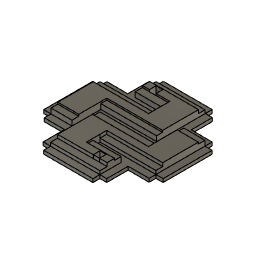
PythonKeyChain (Autodesk Fusion 360 design; units mm, degrees)
Autodesk Fusion 360 part; units mm, degrees
sketch "pythonSketch" plane through (0, 0, 0) normal (0, 0, 1) x (1, 0, 0)
  line L0 (12.2612, -2.5668) -> (26.7, -2.5668)
  line L1 (26.7, -2.5668) -> (26.7, -4.6)
  line L2 (26.7, -4.6) -> (28.8, -4.6)
  line L3 (28.8, -4.6) -> (28.8, -10.8729)
  line L4 (28.8, -10.8729) -> (35, -10.8729)
  line L5 (35, -10.8729) -> (35, -13)
  line L6 (35, -13) -> (37.1372, -13)
  line L7 (37.1372, -13) -> (37.1372, -27.5)
  line L8 (37.1372, -27.5) -> (35, -27.5)
  line L9 (35, -27.5) -> (35, -29.5)
  line L10 (35, -29.5) -> (28.7977, -29.5)
  line L11 (28.7977, -29.5) -> (28.7977, -35.8264)
  line L12 (28.7977, -35.8264) -> (26.777, -35.8264)
  line L13 (26.777, -35.8264) -> (26.777, -37.8923)
  line L14 (26.777, -37.8923) -> (12.2101, -37.8923)
  line L15 (12.2101, -37.8923) -> (12.2101, -35.8264)
  line L16 (12.2101, -35.8264) -> (10, -35.8264)
  line L17 (10, -35.8264) -> (10, -29.5)
  line L18 (10, -29.5) -> (4, -29.5)
  line L19 (4, -29.5) -> (4, -27.5)
  line L20 (4, -27.5) -> (1.8353, -27.5)
  line L21 (1.8353, -27.5) -> (1.8353, -13)
  line L22 (1.8353, -13) -> (4, -13)
  line L23 (4, -13) -> (4, -11)
  line L24 (4, -11) -> (10.1818, -11)
  line L25 (10.1818, -11) -> (10.1818, -4.699)
  line L26 (10.1818, -4.699) -> (12.2719, -4.699)
  line L27 (12.2719, -4.699) -> (12.2612, -2.5668)
  line L28 (20.3394, -10.8945) -> (20.3377, -12.9134)
  line L29 (20.3377, -12.9134) -> (4, -13)
  line L30 (4, -13) -> (4, -27.5)
  line L31 (12.2719, -4.699) -> (26.7, -4.699)
  line L32 (26.7, -4.699) -> (26.7, -19)
  line L33 (26.7, -19) -> (10.2082, -19)
  line L34 (10.2082, -19) -> (10.2082, -27.5)
  line L35 (10.2082, -27.5) -> (4, -27.5)
  line L36 (35, -13) -> (28.7314, -13)
  line L37 (28.7314, -13) -> (28.7314, -21.2454)
  line L38 (28.7314, -21.2454) -> (12.2026, -21.2454)
  line L39 (12.2101, -35.8264) -> (26.777, -35.8264)
  line L40 (26.777, -29.5705) -> (18.4403, -29.5705)
  line L41 (18.4403, -29.5705) -> (18.4403, -27.4588)
  line L42 (18.4403, -27.4588) -> (35, -27.5)
  line L43 (26.777, -29.5705) -> (26.777, -35.8264)
  line L44 (35, -13) -> (35, -27.5)
  line L45 (14.3261, -6.7876) -> (16.303, -6.7893)
  line L46 (16.303, -6.7893) -> (16.3013, -8.805)
  line L47 (16.3013, -8.805) -> (14.3448, -8.8033)
  line L48 (14.3448, -8.8033) -> (14.3261, -6.7876)
  line L49 (22.6655, -31.7169) -> (24.5, -31.7169)
  line L50 (24.5, -31.7169) -> (24.5, -33.682)
  line L51 (24.5, -33.682) -> (22.7033, -33.682)
  line L52 (22.7033, -33.682) -> (22.6655, -31.7169)
  line L53 (12.2703, -6.5992) -> (26.7, -6.5992)
  line L54 (26.7, -4.699) -> (12.2719, -4.699)
  line L55 (4, -15) -> (20.3439, -15)
  line L56 (20.3439, -15) -> (20.3377, -12.9134)
  line L57 (20.3377, -12.9134) -> (4, -13)
  line L58 (4, -13) -> (4, -15)
  line L59 (10.2082, -19) -> (10.2082, -17.2376)
  line L60 (10.2082, -17.2376) -> (26.7, -17.2376)
  line L61 (26.7, -19) -> (10.2082, -19)
  line L62 (26.7, -19) -> (26.7, -17.2376)
  line L63 (4, -25.5) -> (10.2082, -25.5)
  line L64 (10.2082, -25.5) -> (10.2082, -27.5)
  line L65 (10.2082, -27.5) -> (4, -27.5)
  line L66 (4, -27.5) -> (4, -25.5)
  line L67 (28.7314, -14.9455) -> (35, -14.9455)
  line L68 (35, -13) -> (28.7314, -13)
  line L69 (28.7314, -14.9455) -> (35, -14.9455)
  line L70 (12.2063, -23.4679) -> (28.77, -23.4594)
  line L71 (28.77, -23.4594) -> (28.7314, -21.2454)
  line L72 (28.7314, -21.2454) -> (12.2026, -21.2454)
  line L73 (12.2063, -23.4679) -> (12.2026, -21.2454)
  line L74 (18.4403, -27.4588) -> (18.4452, -25.4862)
  line L75 (18.4452, -25.4862) -> (35, -25.4862)
  line L76 (35, -25.4862) -> (35, -27.5)
  line L77 (35, -27.5) -> (18.4403, -27.4588)
  line L78 (18.4403, -29.5705) -> (18.4403, -31.5)
  line L79 (18.4403, -31.5) -> (26.777, -31.5)
  line L80 (26.777, -29.5705) -> (18.4403, -29.5705)
  line L81 (12.2101, -35.8264) -> (12.2101, -33.7534)
  line L82 (26.777, -33.682) -> (26.777, -35.8264)
  line L83 (12.2101, -35.8264) -> (12.2101, -33.7534)
  line L84 (12.2101, -35.8264) -> (12.2101, -33.7534)
  line L85 (12.2101, -33.7534) -> (26.777, -33.682)
  line L86 (26.777, -33.682) -> (26.777, -35.8264)
  line L87 (26.777, -35.8264) -> (12.2101, -35.8264)
  line L88 (12.2063, -23.4679) -> (12.2101, -33.7534)
  line L89 (12.2719, -4.699) -> (12.2703, -6.5992)
  line L90 (12.2666, -10.81) -> (12.2666, -10.8876)
  line L91 (12.2703, -6.5992) -> (12.2666, -10.8876)
  line L92 (20.3394, -10.8945) -> (12.2666, -10.8876)
  line L93 (20.3394, -10.8945) -> (20.3385, -11.904)
  line L94 (12.2684, -8.7434) -> (20.3394, -8.7503)
  line L95 (20.3394, -8.7503) -> (16.3039, -8.7468)
  line L96 (20.3394, -8.7503) -> (20.3394, -10.8945)
  constraint horizontal L0
  constraint perpendicular L0 L1
  constraint perpendicular L1 L2
  constraint perpendicular L2 L3
  constraint perpendicular L1 L4
  constraint perpendicular L4 L5
  constraint perpendicular L5 L6
  constraint perpendicular L6 L7
  constraint perpendicular L7 L8
  constraint perpendicular L8 L9
  constraint perpendicular L9 L10
  constraint perpendicular L10 L11
  constraint perpendicular L11 L12
  constraint perpendicular L12 L13
  constraint perpendicular L13 L14
  constraint perpendicular L12 L15
  constraint perpendicular L15 L16
  constraint perpendicular L16 L17
  constraint perpendicular L17 L18
  constraint perpendicular L16 L19
  constraint perpendicular L17 L20
  constraint perpendicular L20 L21
  constraint perpendicular L17 L22
  constraint perpendicular L22 L23
  constraint perpendicular L23 L24
  constraint perpendicular L22 L25
  constraint perpendicular L25 L26
  constraint perpendicular L20 L30
  constraint perpendicular L1 L31
  constraint perpendicular L31 L32
  constraint perpendicular L1 L33
  constraint perpendicular L33 L34
  constraint perpendicular L19 L35
  constraint perpendicular L5 L36
  constraint perpendicular L36 L37
  constraint perpendicular L5 L38
  constraint perpendicular L13 L39
  constraint perpendicular L13 L40
  constraint perpendicular L40 L41
  constraint perpendicular L12 L43
  constraint perpendicular L8 L44
  constraint perpendicular L45 L46
  constraint perpendicular L46 L47
  constraint horizontal L49
  constraint perpendicular L49 L50
  constraint perpendicular L50 L51
  constraint coincident L32 L53.end
  constraint perpendicular L32 L53
  constraint parallel L31 L54
  constraint coincident L90.start L89
  constraint coincident L30 L55.start
  constraint perpendicular L30 L55
  constraint parallel L29 L57
  constraint perpendicular L33 L59
  constraint coincident L32 L60.end
  constraint perpendicular L32 L60
  constraint coincident L30 L63.start
  constraint coincident L34 L63.end
  constraint perpendicular L34 L63
  constraint coincident L37 L67.start
  constraint coincident L44 L67.end
  constraint perpendicular L44 L67
  constraint parallel L38 L72
  constraint perpendicular L42 L74
  constraint coincident L44 L75.end
  constraint perpendicular L44 L75
  constraint parallel L42 L77
  constraint perpendicular L40 L78
  constraint coincident L43 L79.end
  constraint perpendicular L43 L79
  constraint perpendicular L16 L81
  constraint coincident L43 L82.start
  constraint collinear L89 L90
  constraint perpendicular L90 L92
  constraint perpendicular L92 L93
  constraint midpoint L91 L94.start
  constraint perpendicular L91 L94
  constraint midpoint L94 L95.end
  constraint perpendicular L46 L95
  constraint vertical L96
extrude "Extrude1" add sketch "pythonSketch" along normal blind 3 contours L28 L30 L32 L34 L45 L46 L48 L53 L55 L56 L59 L60 L63 L91 L93 L94 L95 L96 | L37 L41 L43 L44 L67 L69 L70 L71 L74 L75 L78 L79 L85 L88 makes body 1 at (24.5792, -12.2501, 0) makes body 2 at (32.9105, -20.559, 0)
extrude "Extrude2" add sketch "pythonSketch" along normal blind 2.5 contours L46 L47 L48 L90 L91 L92 L94 L95 L96 | L32 L33 L59 L60 L61 L62 | L36 L37 L44 L67 L68 L69 | L30 L34 L35 L63 L64 L65 L66 | L38 L70 L71 L72 L73 | L40 L43 L78 L79 L80 bodies 1 2
extrude "Extrude3" add sketch "pythonSketch" along normal blind 2 contours L31 L32 L53 L54 L89 | L29 L30 L55 L56 L57 L58 | L42 L44 L74 L75 L76 L77 | L39 L43 L81 L82 L83 L84 L85 L86 L87 bodies 1 2
extrude "Extrude4" add sketch "pythonSketch" along normal blind 1 separate body contours L0 L1 L2 L3 L4 L5 L16 L17 L18 L19 L27 L31 L32 L33 L34 L35 L36 L37 L38 L54 L61 L62 L64 L65 L68 L72 L73 L81 L83 L84 L88 | L23 L24 L25 L26 L28 L29 L57 L89 L90 L91 L92 L93 | L20 L21 L22 L30 L58 L66 | L6 L7 L8 L44 L76 | L9 L10 L11 L12 L40 L41 L42 L43 L77 L80 L82 L86 | L13 L14 L15 L39 L87 makes body 3 at (22.5446, -20.4969, 0)
combine "Combine1" operation add target body 2 tool bodies 3 1
named bodies: "python"
